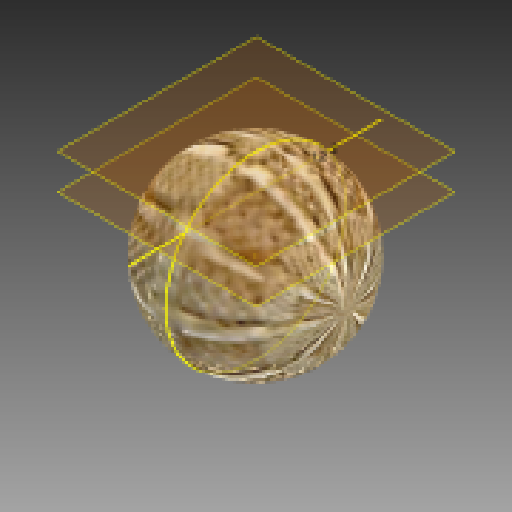
# Autodesk Inventor part: ball
Saved by Autodesk Inventor 2023 (Build 270158000, 158)
## iProperties
Created: 2024-09-29
Part Number: ball
Material: Типовые
Document SubType Name: Modeling
Designer: Ivan
Density: 1 g/cm^3
Appearance: Шотландка — бежевая
Mass: 212.175 g
Surface Area: 172.034 cm^2
Volume: 212.175 cm^3
Author: Ivan
Autodesk Inventor part; units mm, degrees
ref_plane "YZ Plane" through (0, 0, 0) normal (1, 0, 0) x (0, 1, 0)
ref_plane "XY Plane" through (0, 0, 0) normal (0, 0, 1) x (1, 0, 0)
sketch "Эскиз1" plane through (0, 0, 0) normal (0, 1, 0) x (-1, 0, 0)
  arc A0 (37, 0) -> (-37, 0) centre (0, 0) ccw
  line L0 (37, 0) -> (-37, 0)
  dimension "d0" = 37
  constraints: 2 end point, 2 point on circle, 1 centre point, 1 coincident, 1 horizontal
  measures "d0" radius of A0
revolve "Вращение1" add sketch "Эскиз1" angle 360 about axis through (-37, 0, 0) along (1, 0, 0)
ref_plane "РабПлоскость2" through (0, 22.6, 0) normal (0, 1, 0) x (-1, 0, 0)
ref_plane "РабПлоскость1" through (0, 37, 0) normal (0, 1, 0) x (-1, 0, 0)
sketch "Эскиз3" plane through (0, 0, 0) normal (1, 0, 0) x (0, 1, 0)
  circle A0 centre (0, 0) radius 37 projected
  line L0 (22, -29.7489) -> (22, -26.7489)
  line L1 (23.2, -28.8229) -> (23.2, -26.7489)
  line L2 (22, -26.7489) -> (23.2, -26.7489)
  line L3 (22.6, 51.8) -> (22.6, -51.8) projected
  point P0 (22.6, -26.7489)
  dimension "d3" = 3
  dimension "d4" = 1.2
  constraints: 6 end point, 2 point on circle, 2 vertical, 1 horizontal, 1 midpoint, 1 point on line
  measures "d3" distance of L0.start L0.end
  measures "d4" distance of L0.end L1.end
